Autodesk Inventor part; units mm, degrees
(part 2 of 2)
extrude "Extrusion9" cut sketch "Sketch3" against normal blind 5.3 contours A0 | A1 | A4 | A5
ref_plane "Work Plane4" through (-5.09899, -75.436062, 0) normal (0, 0, -1) x (0.7071068, 0.7071068, 0)
extrude "Extrusion10" cut sketch "Sketch3" against normal up to surface (9.3 mm away) contours A0 | A1
sketch "Sketch4" plane through (0, -65.837072, 0) normal (0, -1, 0) x (1, 0, 0)
  line L0 (0, 0) -> (23.1, 0)
  line L1 (0, 0) -> (0, -9.3)
  line L2 (0, -9.3) -> (23.1, -9.3)
  line L3 (23.1, 0) -> (23.1, -9.3)
  line L4 (4, 0) -> (4, -9.3)
  circle A0 centre (20.1, -6.8) radius 3
  circle A1 centre (14.12087, -6.3) radius 3
  circle A2 centre (14.12087, -6.3) radius 2.25
  circle A3 centre (20.1, -6.8) radius 2.5
  line L5 (0, 0) -> (23.1, 0)
  line L6 (11.293146, -9.3) -> (6.793146, -9.3)
  line L7 (6.793146, -9.3) -> (6.793146, 0)
  line L8 (0, -9.3) -> (23.1, -9.3)
  line L9 (23.1, 0) -> (23.1, -9.3)
  circle A4 centre (7, -6.3) radius 3
  dimension "d104" = 4
  dimension "d105" = 6
  dimension "d106" = 6
  dimension "d107" = 4.5
  dimension "d108" = 5
  dimension "d116" = 6
  constraints: 6 tangent, 5 centre point, 4 end point, 3 point on line, 2 coincident, 2 perpendicular
  measures "d104" distance between parallel lines of L1 L4
  measures "d105" diameter of A0
  measures "d106" diameter of A1
  measures "d107" diameter of A2
  measures "d108" diameter of A3
  measures "d116" diameter of A4
hole "Hole1" at (20.1, -65.837072, -6.8) direction (0, 1, 0) diameter 2.459 depth 13.25 thread size "M3x0.5" class "6H" standard "ISO Metric profile"
hole "Hole2" at (7, -65.837072, -6.3) at (14.12087, -65.837072, -6.3) direction (0, 1, 0) diameter 2.459 depth 8 thread size "M3x0.5" class "6H" standard "ISO Metric profile"
sketch "Sketch5" plane through (27.4, 0, -9.3) normal (0, 0, -1) x (-1, 0, 0)
  line L0 (24.9, -17.5) -> (27.4, -17.5)
  line L1 (24.9, -1) -> (24.9, -17.5)
  line L2 (27.4, -1) -> (24.9, -1)
  line L3 (27.4, -17.5) -> (27.4, -65.837072)
  line L4 (0, 0) -> (27.4, 0)
  line L5 (0, -6.5) -> (0, 0)
  line L6 (4.3, -6.5) -> (0, -6.5)
  line L7 (4.3, -65.837072) -> (4.3, -6.5)
  line L8 (27.4, 0) -> (27.4, -1)
  arc A0 (10.623304, -44.239061) -> (10.804346, -51.010357) centre (18.398028, -47.419258) ccw
  arc A1 (23.445574, -40.704923) -> (10.623304, -44.239061) centre (15.05, -35.272213) ccw
  arc A2 (17.69766, -55.79001) -> (23.445574, -40.704923) centre (18.398028, -47.419258) ccw
  arc A3 (10.804346, -51.010357) -> (17.69766, -55.79001) centre (12.7, -55.637072) ccw
  circle A4 centre (7.043146, -49.980218) radius 2.25
  circle A5 centre (18.356854, -61.293926) radius 2.25
  circle A6 centre (7.55, -9.75) radius 3.25
  line L9 (24.9, -6.5) -> (4.3, -6.5)
  line L10 (24.9, -1) -> (24.9, -17.5)
  circle A7 centre (17.55, -9.75) radius 3.25
  line L11 (4.3, -65.837072) -> (4.3, -6.5)
  circle A8 centre (23.4, -24.034887) radius 4
  line L12 (27.4, -17.5) -> (27.4, -65.837072)
  circle A9 centre (23.9, -57.970955) radius 3.5
  circle A10 centre (7.527007, -45.254927) radius 2.5
  arc A11 (23.445574, -40.704923) -> (10.623304, -44.239061) centre (15.05, -35.272213) ccw
  line L13 (4.3, -19.5) -> (24.9, -19.5)
  circle A12 centre (9.424807, -23) radius 3.5
  circle A13 centre (7.527007, -45.254927) radius 3
  line L14 (27.4, -65.837072) -> (4.3, -65.837072)
  point P0 (27.4, 0)
  point P1 (27.4, -15)
  dimension "d124" = 6.5
  dimension "d125" = 6.5
  dimension "d126" = 6.5
  dimension "d127" = 10
  dimension "d128" = 8
  dimension "d129" = 7
  dimension "d130" = 5
  dimension "d133" = 19.5
  dimension "d141" = 7
  dimension "d178" = 6
  constraints: 11 tangent, 7 centre point, 4 end point, 4 point on line, 2 perpendicular, 1 coincident
  measures "d124" diameter of A6
  measures "d125" distance between parallel lines of L4 L9
  measures "d126" diameter of A7
  measures "d127" distance of A6.centre A7.centre
  measures "d128" diameter of A8
  measures "d129" diameter of A9
  measures "d130" diameter of A10
  measures "d133" distance between parallel lines of L13 L4
  measures "d141" diameter of A12
  measures "d178" diameter of A13
hole "Hole3" at (3.5, -57.970955, -9.3) at (4, -24.034887, -9.3) at (19.872993, -45.254927, -9.3) at (19.85, -9.75, -9.3) at (9.85, -9.75, -9.3) at (17.975193, -23, -9.3) direction (0, 0, 1) diameter 2.459 depth 10 thread size "M3x0.5" class "6H" standard "ISO Metric profile"
sketch "Sketch6" plane through (0, -65.837072, 0) normal (-1, 0, 0) x (0, 0, 1)
  line L0 (0, 40.042024) -> (0, 20.295048)
  line L1 (2, 18.6) -> (2, 42.737072)
  line L2 (0, 40.042024) -> (3.8, 40.042024)
  circle A0 centre (1.9, 30.668536) radius 1.0065
  line L3 (0, 20.295048) -> (3.8, 20.295048)
  line L4 (3.8, 40.042024) -> (3.8, 20.295048)
  point P0 (0, 65.837072)
  point P1 (1.9, 30.668536)
  constraints: 2 end point, 1 coincident
hole "Hole4" at (0, -35.168536, 1.9) direction (1, 0, 0) diameter 2.9 end through all countersink diameter 7 countersink angle 90 clearance for "Countersunk Flat Head Screw ISO 2009/7046" size "M2.5" standard "ISO"
sketch "Sketch8" plane through (27.4, -6.5, -9.3) normal (1, 0, 0) x (0, 0, -1)
  line L0 (-5.3, 0) -> (0, 0)
  line L1 (0, 0) -> (0, 6.5)
  line L2 (-9.3, 6.5) -> (0, 6.5)
  line L3 (-9.3, 0.598313) -> (-9.3, 6.5)
  line L4 (-5.3, 0) -> (0, 6.5)
  line L5 (-5.3, 0.598313) -> (-5.3, 0)
  line L6 (-9.3, 0.598313) -> (-5.3, 0.598313)
  line L7 (0, 0) -> (-3.183466, 2.595749)
  point P0 (-9.3, 6.5)
  point P1 (-2.65, 3.25)
  constraints: 4 end point, 1 midpoint, 1 perpendicular, 1 point on line
hole "Hole6" at (27.4, -3.25, -6.65) direction (-1, 0, 0) diameter 2.459 depth 8 thread size "M3x0.5" class "6H" standard "ISO Metric profile"
sketch "Sketch9" plane through (23.1, -65.837072, -9.3) normal (1, 0, 0) x (0, 0, -1)
  line L0 (-9.3, 0) -> (-9.3, 43.400579)
  line L1 (-5.3, 57.62504) -> (-9.3, 57.62504)
  line L2 (-9.3, 0) -> (-9.3, 43.400579)
  line L3 (-9.3, 0) -> (0, 0)
  line L4 (0, 0) -> (0, 59.337072)
  line L5 (-5.3, 59.337072) -> (0, 59.337072)
  line L6 (-5.3, 59.337072) -> (-5.3, 57.62504)
  circle A0 centre (-3.3, 52.213573) radius 2.5
  circle A1 centre (-6.55, 2.75) radius 2.75
  circle A2 centre (-3.3, 52.213573) radius 2
  line L7 (-5.3, 46.137072) -> (-5.3, 56.137072)
  line L8 (-5.3, 43.400579) -> (-9.3, 43.400579)
  line L9 (-5.3, 57.62504) -> (-9.3, 57.62504)
  line L10 (-9.3, 48.394682) -> (-9.3, 57.62504)
  line L11 (-9.3, 48.394682) -> (-5.3, 48.394682)
  line L12 (-5.3, 48.394682) -> (-5.3, 43.400579)
  point P0 (-9.3, 65.837072)
  point P1 (-5.3, 47.634782)
  point P2 (-4, 54.087072)
  point P3 (-9.3, 36.437072)
  dimension "d174" = 4
  dimension "d165" = 5
  dimension "d173" = 5.5
  constraints: 2 centre point, 2 tangent, 1 coincident, 1 vertical, 3 other
  measures "d165" diameter of A0
  measures "d173" diameter of A1
hole "Hole7" at (23.1, -13.623499, -6) at (23.1, -63.087072, -2.75) direction (-1, 0, 0) diameter 2.013 depth 10 thread size "M2.5x0.45" class "6H" standard "ISO Metric profile"
fillet "Fillet1" radius 1 6 edges at (20.9375, -21.188, -2) (8.4625, -8.212, -2) (4.4609, -5.9017, -2) (3, -7.965, -2) (3, -10.8318, -2) (5.9625, -12.5422, -2)
hole "Hole8" at (1.4, -40.269072, -9.3) at (1.4, -29.025192, -9.3) direction (0, 0, 1) diameter 1.4 end through all
sketch "Sketch12" plane through (2.5, -17.5, 0) normal (-1, 0, 0) x (0, 0, 1)
  circle A0 centre (-6, 10) radius 1.25 projected
  point P0 (0, 17.5)
hole "Hole9" at (2.5, -7.5, -6) direction (1, 0, 0) diameter 2.013 depth 10 thread size "M2.5x0.45" class "6H" standard "ISO Metric profile"
sketch "Sketch13" plane through (0, 0, -3.1) normal (0, 0, -1) x (-1, 0, 0)
  circle A0 centre (-14.7, -55.637072) radius 14
  circle A1 centre (-14.7, -14.7) radius 14
  arc A2 (-3.954426, -40.704923) -> (-16.776696, -44.239061) centre (-12.35, -35.272213) ccw
  arc A3 (-6.63248, -43.476478) -> (-13.056865, -45.247199) centre (-12.35, -35.272213) ccw
  circle A4 centre (-18.490592, -39.578386) radius 2.5
  circle A5 centre (-18.362153, -30.788463) radius 2.5
  circle A6 centre (-7.503908, -29.548106) radius 2.5
  circle A7 centre (-6.050082, -39.341737) radius 2.5
  circle A8 centre (-9.001972, -47.419258) radius 4.6
  point P0 (0, 0)
  point P1 (-19.483471, -42.280322)
  dimension "d206" = 5
  dimension "d207" = 5
  dimension "d215" = 5
  dimension "d216" = 5
  dimension "d218" = 1.5
  constraints: 7 tangent, 4 centre point
  measures "d206" diameter of A4
  measures "d207" diameter of A5
  measures "d215" diameter of A6
  measures "d216" diameter of A7
hole "Hole10" at (18.490592, -39.578386, -3.1) at (18.362153, -30.788463, -3.1) at (7.503908, -29.548106, -3.1) at (6.050082, -39.341737, -3.1) direction (0, 0, 1) diameter 2.7 end through all counterbore diameter 5 counterbore depth 1.1 clearance for "Countersunk Flat Head Screw ISO 2009/7046" size "M2.5" standard "ISO"
sketch "Sketch14" plane through (0, 0, -3.1) normal (0, 0, -1) x (-1, 0, 0)
  arc A0 (-8.150054, -37.985229) -> (-3.950109, -40.698245) centre (-6.050082, -39.341737) ccw
  arc A1 (-16.443728, -38.142995) -> (-8.150054, -37.985229) centre (-12.35, -35.272213) ccw
  arc A2 (-20.537456, -41.013777) -> (-16.443728, -38.142995) centre (-18.490592, -39.578386) ccw
  arc A3 (-20.537456, -41.013777) -> (-13.056865, -45.247199) centre (-12.35, -35.272213) ccw
  arc A4 (-6.63248, -43.476478) -> (-13.056865, -45.247199) centre (-9.001972, -47.419258) ccw
  arc A5 (-6.63248, -43.476478) -> (-3.950109, -40.698245) centre (-12.35, -35.272213) ccw
  arc A6 (-20.366204, -29.293879) -> (-16.358102, -32.283046) centre (-18.362153, -30.788463) ccw
  arc A7 (-20.366204, -29.293879) -> (-20.537456, -41.013777) centre (-12.35, -35.272213) ccw
  arc A8 (-16.443728, -38.142995) -> (-20.537456, -41.013777) centre (-18.490592, -39.578386) ccw
  arc A9 (-16.358102, -32.283046) -> (-16.443728, -38.142995) centre (-12.35, -35.272213) ccw
  arc A10 (-5.888544, -27.640071) -> (-9.119272, -31.456142) centre (-7.503908, -29.548106) ccw
  arc A11 (-5.888544, -27.640071) -> (-20.366204, -29.293879) centre (-12.35, -35.272213) ccw
  arc A12 (-16.358102, -32.283046) -> (-20.366204, -29.293879) centre (-18.362153, -30.788463) ccw
  arc A13 (-9.119272, -31.456142) -> (-16.358102, -32.283046) centre (-12.35, -35.272213) ccw
  arc A14 (-3.950109, -40.698245) -> (-8.150054, -37.985229) centre (-6.050082, -39.341737) ccw
  arc A15 (-3.950109, -40.698245) -> (-5.888544, -27.640071) centre (-12.35, -35.272213) ccw
  arc A16 (-9.119272, -31.456142) -> (-5.888544, -27.640071) centre (-7.503908, -29.548106) ccw
  arc A17 (-8.150054, -37.985229) -> (-9.119272, -31.456142) centre (-12.35, -35.272213) ccw
  line L0 (-16.455005, -41.029724) -> (-15.252677, -39.343388)
  arc A18 (-20.537456, -41.013777) -> (-16.443728, -38.142995) centre (-18.490592, -39.578386) ccw
  line L1 (-9.841276, -28.661138) -> (-10.576064, -30.597477)
  line L2 (-6.24345, -31.707098) -> (-8.032017, -32.751296)
  line L3 (-5.163114, -37.004369) -> (-7.426827, -36.145351)
  line L4 (-8.029001, -40.869441) -> (-9.294592, -39.230051)
  line L5 (-19.161604, -37.17012) -> (-17.166531, -36.614236)
  line L6 (-19.103243, -33.176095) -> (-17.125264, -33.790033)
  line L7 (-16.28503, -29.39722) -> (-15.132486, -31.117965)
  arc A19 (-5.888544, -27.640071) -> (-9.119272, -31.456142) centre (-7.503908, -29.548106) ccw
  arc A20 (-8.150054, -37.985229) -> (-3.950109, -40.698245) centre (-6.050082, -39.341737) ccw
  arc A21 (-3.950109, -40.698245) -> (-8.150054, -37.985229) centre (-6.050082, -39.341737) ccw
  point P0 (0, 0)
  point P1 (-16.28503, -29.39722)
  point P2 (-16.443728, -38.142995)
  point P3 (-16.443728, -38.142995)
  point P4 (-16.443728, -38.142995)
  point P5 (-16.443728, -38.142995)
  point P6 (-16.358102, -32.283046)
  point P7 (-16.358102, -32.283046)
  point P8 (-16.358102, -32.283046)
  point P9 (-16.358102, -32.283046)
  point P10 (-9.119272, -31.456142)
  point P11 (-9.119272, -31.456142)
  point P12 (-9.119272, -31.456142)
  point P13 (-9.119272, -31.456142)
  point P14 (-8.150054, -37.985229)
  point P15 (-8.150054, -37.985229)
  point P16 (-8.150054, -37.985229)
  point P17 (-8.150054, -37.985229)
  constraints: 17 point on circle, 16 end point, 9 tangent, 7 line through centre, 1 coincident, 1 perpendicular, 3 other
extrude "Extrusion12" cut sketch "Sketch14" against normal up to surface (1.1 mm away) contours A0 L4 A1 | A17 L3 A14 | L0 A2 A1 | A17 A16 L2 | A8 L5 A9 | A13 L1 A10 | A6 A9 L6 | L7 A13 A12
sketch "Sketch15" plane through (0, 0, 0) normal (0, 1, 0) x (1, 0, 0)
  line L0 (27.4, 0) -> (0, 0) projected
  line L1 (27.4, 0) -> (27.4, 9.3) projected
  line L2 (27.4, 9.3) -> (0, 9.3) projected
  line L3 (0, 0) -> (0, 9.3) projected
  line L4 (2.5, 9.3) -> (17.4, 9.3)
  line L5 (3, 9.3) -> (3, 0)
  line L6 (23.1, 9.3) -> (23.1, 0)
  line L7 (23.1, 4) -> (3, 4)
  line L8 (13.05, 0) -> (13.05, 4)
  circle A0 centre (18.075, 3) radius 3
  circle A1 centre (8.025, 3) radius 3
  line L9 (27.4, 0) -> (0, 0) projected
  dimension "d224" = 3
  dimension "d225" = 4.3
  dimension "d226" = 4
  dimension "d227" = 6
  dimension "d228" = 6
  dimension "d229" = 5.025
  dimension "d230" = 5.025
  dimension "d231" = 5.025
  dimension "d232" = 5.025
  constraints: 10 end point, 8 point on line, 4 perpendicular, 2 centre point, 2 midpoint, 2 tangent, 1 horizontal
  measures "d224" distance between parallel lines of L3 L5
  measures "d225" distance between parallel lines of L1 L6
  measures "d226" distance between parallel lines of L0 L7
  measures "d227" diameter of A0
  measures "d228" diameter of A1
  measures "d229" distance from line of L8 A1.centre
  measures "d230" distance from line of A1.centre L5
  measures "d231" distance from line of A0.centre L8
  measures "d232" distance from line of L6 A0.centre
hole "Hole11" at (18.075, 0, -3) at (8.025, 0, -3) direction (0, -1, 0) diameter 2.85 depth 8.212032 thread size "M3.5x0.6" class "6H" standard "ISO Metric profile"
ref_plane "Work Plane5" through (0, 1, 0) normal (0, 1, 0) x (1, 0, 0)
sketch "Sketch16" plane through (0, 1, 0) normal (0, 1, 0) x (1, 0, 0)
  circle A0 centre (18.075, 3) radius 1.425 projected
  circle A1 centre (8.025, 3) radius 1.425 projected
  point P0 (0, 0)
hole "Hole12" at (18.075, 1, -3) at (8.025, 1, -3) direction (0, -1, 0) diameter 0.1 depth 5 countersink diameter 7 countersink angle 90
fillet "Fillet2" radius 1 8 edges at (15.2527, -39.3434, -2.55) (17.1665, -36.6142, -2.55) (17.1253, -33.79, -2.55) (15.1325, -31.118, -2.55) (10.5761, -30.5975, -2.55) (8.032, -32.7513, -2.55) (7.4268, -36.1454, -2.55) (9.2946, -39.2301, -2.55)
body "Solid1"
